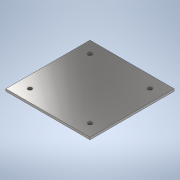
# Autodesk Inventor part: 21015-22-1-1- Floor Plate
Saved by Autodesk Inventor 2022 (Build 260153000, 153)
## iProperties
Created: 2021-06-17
Part Number: 21015-22-1-1- Floor Plate
Material: Steel, Carbon
Document SubType Name: Modeling
Designer: Skynet
Density: 7.85 g/cm^3
Appearance: Semi-Polished
Author: Skynet
Autodesk Inventor part; units mm, degrees
ref_plane "YZ Plane" through (0, 0, 0) normal (1, 0, 0) x (0, 1, 0)
ref_plane "XZ Plane" through (0, 0, 0) normal (0, 1, 0) x (-1, 0, 0)
ref_plane "XY Plane" through (0, 0, 0) normal (0, 0, 1) x (1, 0, 0)
sketch "Sketch1" plane through (0, 0, 0) normal (0, 1, 0) x (-1, 0, 0)
  line L0 (0, 0) -> (355.6, 0)
  line L1 (355.6, 0) -> (355.6, -355.6)
  line L2 (355.6, -355.6) -> (0, -355.6)
  line L3 (0, -355.6) -> (0, 0)
  circle A0 centre (304.8, -304.8) radius 8.3312
  circle A1 centre (304.8, -50.8) radius 8.3312
  circle A2 centre (50.8, -304.8) radius 8.3312
  circle A3 centre (50.8, -50.8) radius 8.3312
  dimension "d0" = 355.6
  dimension "d1" = 355.6
  dimension "d2" = 16.6624
  dimension "d3" = 50.8
  dimension "d4" = 50.8
  constraints: 8 end point, 4 centre point, 2 parallel, 1 horizontal, 1 perpendicular
  measures "d0" distance of L0.end L1.end
  measures "d1" distance of L1.end L2.end
  measures "d2" diameter of A0
  measures "d3" distance from line of L2 A0.centre
  measures "d4" distance from line of A0.centre L1
extrude "Extrusion1" add sketch "Sketch1" along normal blind 9.525
body "Solid1"
